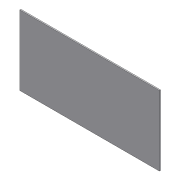
# Autodesk Inventor part: GE-12028-02
Saved by Autodesk Inventor 2012 (Build 160160000, 160)
## iProperties
Created: 2008-05-29
Part Number: GE-12028-02
Document SubType Name: Modeling
Designer: narosenberg
Density: 1 g/cm^3
Description: Plate, Stop
Mass: 262.193 g
Surface Area: 1690.32 cm^2
Volume: 262.193 cm^3
Material: Default
Author: narosenberg
Autodesk Inventor part; units mm, degrees
ref_plane "YZ Plane" through (0, 0, 0) normal (1, 0, 0) x (0, 1, 0)
ref_plane "XZ Plane" through (0, 0, 0) normal (0, 1, 0) x (-1, 0, 0)
ref_plane "XY Plane" through (0, 0, 0) normal (0, 0, 1) x (1, 0, 0)
sketch "Sketch1" plane through (0, 0, 0) normal (0, 0, 1) x (1, 0, 0)
  line L0 (-35.9524, 179.3111) -> (370.4476, 179.3111)
  line L1 (370.4476, 179.3111) -> (370.4476, -23.8889)
  line L2 (370.4476, -23.8889) -> (-35.9524, -23.8889)
  line L3 (-35.9524, -23.8889) -> (-35.9524, 179.3111)
  dimension "d0" = 406.4
  dimension "d1" = 203.2
  constraints: 8 end point, 2 parallel, 1 horizontal, 1 perpendicular
  measures "d0" distance of L0.start L0.end
  measures "d1" distance between parallel lines of L2 L0
extrude "Extrusion1" add sketch "Sketch1" along normal blind 3.175
body "Solid1"
